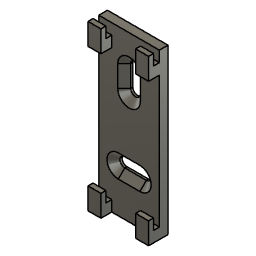
mountplate (Autodesk Fusion 360 design; units mm, degrees)
Autodesk Fusion 360 part; units mm, degrees
sketch "Skizze2" plane through (0, 0, 0) normal (0, 0, 1) x (1, 0, 0)
  line L0 (0, 0) -> (28.074, 0)
  line L1 (28.074, 0) -> (28.074, 76)
  line L2 (28.074, 76) -> (0, 76)
  line L3 (0, 76) -> (0, 0)
  line L4 (0, 76) -> (6, 76)
  line L5 (6, 76) -> (6, 66)
  line L6 (6, 66) -> (0, 66)
  line L7 (0, 66) -> (0, 76)
  line L8 (28.074, 76) -> (22.074, 76)
  line L9 (22.074, 76) -> (22.074, 66)
  line L10 (22.074, 66) -> (28.074, 66)
  line L11 (28.074, 66) -> (28.074, 76)
  line L12 (0, 0) -> (6, 0)
  line L13 (6, 0) -> (6, 10)
  line L14 (6, 10) -> (0, 10)
  line L15 (0, 10) -> (0, 0)
  line L16 (28.074, 0) -> (22.074, 0)
  line L17 (22.074, 0) -> (22.074, 10)
  line L18 (22.074, 10) -> (28.074, 10)
  line L19 (28.074, 10) -> (28.074, 0)
  line L20 (14.037, 76) -> (14.037, 0) construction
  line L21 (0, 20) -> (28.074, 20) construction
  line L22 (0, 56) -> (28.074, 56) construction
  circle A0 centre (14.037, 61) radius 2.25
  circle A1 centre (14.037, 51) radius 2.25
  circle A2 centre (9.037, 20) radius 2.25
  circle A3 centre (19.037, 20) radius 2.25
  line L23 (11.787, 61) -> (11.787, 51)
  line L24 (16.287, 61) -> (16.287, 51)
  line L25 (9.037, 22.25) -> (19.037, 22.25)
  line L26 (9.037, 17.75) -> (19.037, 17.75)
  line L27 (0, 76) -> (6, 76)
  line L28 (6, 76) -> (6, 71)
  line L29 (6, 71) -> (0, 71)
  line L30 (0, 71) -> (0, 76)
  line L31 (22.074, 76) -> (28.074, 76)
  line L32 (28.074, 76) -> (28.074, 71)
  line L33 (28.074, 71) -> (22.074, 71)
  line L34 (22.074, 71) -> (22.074, 76)
  line L35 (0, 10) -> (6, 10)
  line L36 (6, 10) -> (6, 5)
  line L37 (6, 5) -> (0, 5)
  line L38 (0, 5) -> (0, 10)
  line L39 (22.074, 10) -> (28.074, 10)
  line L40 (28.074, 10) -> (28.074, 5)
  line L41 (28.074, 5) -> (22.074, 5)
  line L42 (22.074, 5) -> (22.074, 10)
  point P0 (14.037, 61)
  point P1 (14.037, 51)
  point P2 (9.037, 20)
  point P3 (19.037, 20)
  point P4 (14.037, 56)
  point P5 (14.037, 20)
  dimension "d1" = 28.074
  dimension "d2" = 76
  dimension "d3" = 6
  dimension "d4" = 10
  dimension "d5" = 6
  dimension "d6" = 10
  dimension "d7" = 6
  dimension "d8" = 10
  dimension "d9" = 6
  dimension "d10" = 10
  dimension "d11" = 20
  dimension "d12" = 20
  dimension "d13" = 5
  dimension "d14" = 5
  dimension "d15" = 5
  dimension "d16" = 5
  dimension "d17" = 4.5
  dimension "d18" = 4.5
  dimension "d19" = 4.5
  dimension "d20" = 4.5
  dimension "d23" = 5
  constraint horizontal L0
  constraint vertical L1
  constraint horizontal L2
  constraint vertical L3
  constraint coincident L0.start L3.end
  constraint horizontal L4
  constraint vertical L5
  constraint horizontal L6
  constraint vertical L7
  constraint horizontal L8
  constraint vertical L9
  constraint horizontal L10
  constraint vertical L11
  constraint horizontal L12
  constraint vertical L13
  constraint horizontal L14
  constraint vertical L15
  constraint horizontal L16
  constraint vertical L17
  constraint horizontal L18
  constraint vertical L19
  constraint midpoint L2 L20.start
  constraint midpoint L0 L20.end
  constraint coincident L3 L21.start
  constraint coincident L1 L21.end
  constraint perpendicular L1 L21
  constraint coincident L3 L22.start
  constraint coincident L1 L22.end
  constraint perpendicular L1 L22
  constraint coincident L20 P0
  constraint coincident L20 P1
  constraint coincident L21 P2
  constraint coincident L21 P3
  constraint midpoint L22 P4
  constraint midpoint L21 P5
  constraint coincident P0 A0.centre
  constraint coincident P1 A1.centre
  constraint coincident P2 A2.centre
  constraint coincident P3 A3.centre
  constraint coincident A0 L23.start
  constraint coincident A1 L23.end
  constraint coincident A0 L24.start
  constraint coincident A1 L24.end
  constraint parallel L23 L24
  constraint coincident A2 L25.start
  constraint coincident A3 L25.end
  constraint coincident A2 L26.start
  constraint coincident A3 L26.end
  constraint parallel L25 L26
  constraint tangent A0 L23
  constraint tangent A0 L24
  constraint tangent A2 L25
  constraint tangent A2 L26
  constraint horizontal L27
  constraint vertical L28
  constraint horizontal L29
  constraint vertical L30
  constraint horizontal L31
  constraint vertical L32
  constraint horizontal L33
  constraint vertical L34
  constraint midpoint L11 L32.end
  constraint horizontal L35
  constraint vertical L36
  constraint horizontal L37
  constraint vertical L38
  constraint midpoint L13 L36.end
  constraint horizontal L39
  constraint vertical L40
  constraint horizontal L41
  constraint vertical L42
  constraint midpoint L19 L40.end
  measures "d1" distance of L0.start L0.end
  measures "d2" distance of L0.start L2.end
  measures "d3" distance of L2.end L4.end
  measures "d4" distance of L2.end L6.end
  measures "d5" distance of L1.end L8.end
  measures "d6" distance of L1.end L10.end
  measures "d7" distance of L0.start L12.end
  measures "d8" distance of L0.start L14.end
  measures "d9" distance of L0.end L16.end
  measures "d10" distance of L0.end L18.end
  measures "d11" distance of L2 L22
  measures "d12" distance of L0 L21
  measures "d13" distance of P0 P4
  measures "d14" distance of P1 P4
  measures "d15" distance of P2 P5
  measures "d16" distance of P3 P5
  measures "d17" diameter of A0
  measures "d18" diameter of A1
  measures "d19" diameter of A2
  measures "d20" diameter of A3
  measures "d23" distance of L2.end L29.end
extrude "Extrusion1" add sketch "Skizze2" along normal blind 4 contours L0 L1 L2 L3 L5 L6 L9 L10 L13 L14 L17 L18 L28 L34 L35 L36 L39 L42
extrude "Extrusion2" add sketch "Skizze2" along normal blind 9 contours L0 L3 L12 L13 L15 L37 | L3 L13 L14 L15 L35 L36 L37 L38 | L0 L1 L16 L17 L19 L41 | L1 L17 L18 L19 L39 L40 L41 L42 | L3 L5 L6 L7 L29 | L2 L3 L4 L5 L7 L27 L28 L29 L30 | L1 L9 L10 L11 L33 | L1 L2 L8 L9 L11 L31 L32 L33 L34
extrude "Extrusion3" cut sketch "Skizze2" along normal blind 6.7 contours L3 L13 L14 L15 L35 L36 L37 L38 | L1 L17 L18 L19 L39 L40 L41 L42 | L2 L3 L4 L5 L7 L27 L28 L29 L30 | L1 L2 L8 L9 L11 L31 L32 L33 L34
extrude "Extrusion4" add sketch "Skizze2" along normal blind 4 contours L3 L13 L14 L15 L35 L36 L37 L38 | L1 L17 L18 L19 L39 L40 L41 L42 | L2 L3 L4 L5 L7 L27 L28 L29 L30 | L1 L2 L8 L9 L11 L31 L32 L33 L34
chamfer "Fase1" distance 3 angle 45 8 edges at (14.037, 63.25, 4) (16.287, 56, 4) (14.037, 48.75, 4) (11.787, 56, 4) (14.037, 22.25, 4) (21.287, 20, 4) (14.037, 17.75, 4) (6.787, 20, 4)
